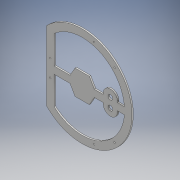
# Autodesk Inventor part: Top Plate1
Saved by Autodesk Inventor 2018 (Build 220112000, 112)
## iProperties
Created: 2017-10-19
Part Number: Top Plate1
Material: Generic
Document SubType Name: Modeling
Designer: BrisbaneMatt
Density: 1 g/cm^3
Appearance: Default
Author: BrisbaneMatt
Autodesk Inventor part; units mm, degrees
ref_plane "YZ Plane" through (0, 0, 0) normal (1, 0, 0) x (0, 1, 0)
ref_plane "XZ Plane" through (0, 0, 0) normal (0, 1, 0) x (-1, 0, 0)
ref_plane "XY Plane" through (0, 0, 0) normal (0, 0, 1) x (1, 0, 0)
sketch "Sketch1" plane through (0, 0, 0) normal (0, 1, 0) x (-1, 0, 0)
  circle A0 centre (0, 0) radius 105
  line L0 (105, 0) -> (75, 0)
  line L1 (75, 0) -> (75, -73.4847)
  line L2 (75, 0) -> (75, 73.4847)
  dimension "d0" = 210
  dimension "d1" = 30
  constraints: 6 end point, 3 point on circle, 1 centre point, 1 coincident, 1 horizontal, 1 perpendicular, 1 point on line
  measures "d0" diameter of A0
  measures "d1" distance of L0.start L0.end
extrude "Extrusion1" add sketch "Sketch1" along normal blind 3 contours L2 L1 A0
sketch "Sketch2" plane through (0, 3, 0) normal (0, 1, 0) x (1, 0, 0)
  line L0 (-75, 73.4847) -> (-75, -73.4847) projected
  line L1 (-75, 0) -> (-67.25, 0)
  line L2 (-67.25, 0) -> (-67.25, -52.6096)
  line L3 (-67.25, -52.6096) -> (-67.25, 59.9001)
  line L4 (0, 0) -> (-67.25, -18.0196)
  line L5 (0, 0) -> (69.6223, 0) construction
  line L6 (0, 0) -> (-67.25, 18.0196)
  line L7 (0, 0) -> (69.6223, 0) construction
  line L8 (0, 0) -> (25.0407, -93.4533)
  line L9 (0, 0) -> (96.75, 0) construction
  line L10 (0, 0) -> (68.4126, -68.4126)
  line L11 (0, 0) -> (96.75, 0) construction
  line L12 (0, 0) -> (25.0407, 93.4533)
  line L13 (0, 0) -> (96.75, 0) construction
  line L14 (0, 0) -> (68.4126, 68.4126)
  line L15 (0, 0) -> (96.75, 0) construction
  circle A0 centre (-67.25, 18.0196) radius 1.5
  circle A1 centre (-67.25, -18.0196) radius 1.5
  circle A2 centre (25.0407, 93.4533) radius 1.5
  circle A3 centre (68.4126, 68.4126) radius 1.5
  circle A4 centre (68.4126, -68.4126) radius 1.5
  circle A5 centre (25.0407, -93.4533) radius 1.5
  dimension "d4" = 7.75
  dimension "d5" = 165
  dimension "d6" = 165
  dimension "d7" = 96.75
  dimension "d8" = 75
  dimension "d9" = 96.75
  dimension "d10" = 45
  dimension "d11" = 96.75
  dimension "d12" = 75
  dimension "d13" = 96.75
  dimension "d14" = 45
  dimension "d15" = 3
  dimension "d16" = 3
  dimension "d17" = 3
  dimension "d18" = 3
  dimension "d19" = 3
  dimension "d20" = 3
  constraints: 30 end point, 7 horizontal, 6 centre point, 6 coincident, 6 equal length, 3 perpendicular, 3 point on line, 1 midpoint
  measures "d4" distance of L1.start L1.end
  measures "d5" angle of L4 L5
  measures "d6" angle of L7 L6
  measures "d7" distance of L4.start L8.end
  measures "d8" angle of L8 L9
  measures "d9" distance of L4.start L10.end
  measures "d10" angle of L10 L11
  measures "d11" distance of L4.start L12.end
  measures "d12" angle of L13 L12
  measures "d13" distance of L4.start L14.end
  measures "d14" angle of L15 L14
  measures "d15" diameter of A0
  measures "d16" diameter of A1
  measures "d17" diameter of A2
  measures "d18" diameter of A3
  measures "d19" diameter of A4
  measures "d20" diameter of A5
extrude "Extrusion2" cut sketch "Sketch2" against normal blind 3 contours A1 L4 L2 | L2 A1 | A0 L3 | L3 L6 A0 | L4 A1 L2 | L3 A0 L6 | A2 | A3 | A4 | A5
sketch "Sketch3" plane through (0, 3, 0) normal (0, 1, 0) x (1, 0, 0)
  circle A0 centre (-67.25, -18.0196) radius 1.5 projected
  line L0 (-67.25, -18.0196) -> (-75, -18.0196)
  line L1 (-75, 73.4847) -> (-75, -73.4847) projected
  line L2 (-75, -18.0196) -> (-59.5, -18.0196)
  line L3 (-59.5, -18.0196) -> (-59.5, -66.8581)
  line L4 (-59.5, -18.0196) -> (-59.5, 66.8581)
  arc A1 (-59.5, -66.8581) -> (-59.5, 66.8581) centre (0, 0) ccw
  point P0 (0, 0)
  dimension "d23" = 15.5
  constraints: 8 end point, 3 point on line, 2 point on circle, 1 centre point, 1 horizontal, 1 vertical
  measures "d23" distance of L0.end L2.end
extrude "Extrusion3" cut sketch "Sketch3" against normal blind 3 contours L4 A1 L3
sketch "Sketch4" plane through (0, 3, 0) normal (0, 1, 0) x (1, 0, 0)
  arc A0 (-59.5, -66.8581) -> (-59.5, 66.8581) centre (0, 0) ccw projected
  line L0 (89.5, 0) -> (59.5, 0)
  line L1 (59.5, 0) -> (59.5, 10)
  line L2 (59.5, 10) -> (59.5, -10)
  circle A1 centre (59.5, -10) radius 5
  circle A2 centre (59.5, 10) radius 5
  circle A3 centre (59.5, 10) radius 15
  circle A4 centre (59.5, -10) radius 15
  line L3 (44.5, -10) -> (44.5, 10)
  line L4 (74.5, 10) -> (74.5, -10)
  point P0 (0, 0)
  dimension "d27" = 30
  dimension "d28" = 10
  dimension "d29" = 20
  dimension "d30" = 10
  dimension "d31" = 10
  constraints: 10 end point, 5 point on circle, 4 centre point, 4 coincident, 2 tangent, 1 horizontal, 1 parallel, 1 perpendicular, 1 point on line, 1 vertical
  measures "d27" distance of L0.start L0.end
  measures "d28" distance of L0.end L1.end
  measures "d29" distance of L1.end L2.end
  measures "d30" diameter of A1
  measures "d31" diameter of A2
extrude "Extrusion4" add sketch "Sketch4" against normal blind 3
sketch "Sketch5" plane through (0, 3, 0) normal (0, 1, 0) x (1, 0, 0)
  line L0 (44.5, -10) -> (44.5, 10) projected
  line L1 (44.5, 0) -> (-59.5, 0)
  line L2 (-59.5, 66.8581) -> (-59.5, -66.8581) projected
  line L3 (-41.4459, 0) -> (-41.4459, 7.5)
  line L4 (-41.4459, 7.5) -> (-41.4459, -7.5)
  line L5 (-41.4459, -7.5) -> (-59.5, -7.5)
  line L6 (-41.4459, -7.5) -> (44.5, -7.5)
  line L7 (-41.4459, 7.5) -> (-59.5, 7.5)
  line L8 (-41.4459, 7.5) -> (44.5, 7.5)
  point P0 (0, 0)
  dimension "d34" = 7.5
  dimension "d35" = 15
  constraints: 14 end point, 7 point on line, 3 perpendicular, 2 midpoint
  measures "d34" distance of L3.start L3.end
  measures "d35" distance of L3.end L4.end
extrude "Extrusion5" add sketch "Sketch5" against normal blind 3 contours L1 L3 L8 L0 | L5 L2 L1 L4 | L1 L2 L7 L3
sketch "Sketch6" plane through (0, 3, 0) normal (0, 1, 0) x (1, 0, 0)
  line L0 (-41.4459, -7.5) -> (-41.4459, 0) projected
  line L1 (-41.4459, 0) -> (44.5, 0) projected
  line L2 (-41.4459, -7.5) -> (44.5, -7.5)
  line L3 (44.5, -7.5) -> (44.5, 0)
  line L4 (44.5, 0) -> (-41.4459, 0)
  line L5 (-41.4459, 0) -> (-41.4459, -7.5)
  point P0 (0, 0)
  constraints: 8 end point, 2 parallel, 1 horizontal, 1 perpendicular
extrude "Extrusion6" add sketch "Sketch6" against normal blind 3
sketch "Sketch7" plane through (0, 3, 0) normal (0, 1, 0) x (1, 0, 0)
  line L0 (44.5, -7.5) -> (-59.5, -7.5) projected
  line L1 (74.5, 10) -> (74.5, -10) projected
  line L2 (44.5, -7.5) -> (74.5, -7.5)
  line L3 (74.5, -7.5) -> (74.5, 7.5)
  line L4 (74.5, 7.5) -> (44.5, 7.5)
  line L5 (44.5, 7.5) -> (44.5, -7.5)
  line L6 (74.5, 7.5) -> (92.1337, 7.5)
  line L7 (92.1337, 7.5) -> (92.1337, -7.5)
  line L8 (92.1337, -7.5) -> (74.5, -7.5)
  line L9 (74.5, -7.5) -> (74.5, 7.5)
  point P0 (0, 0)
  dimension "d40" = 15
  constraints: 16 end point, 4 parallel, 2 horizontal, 2 perpendicular, 2 point on line
  measures "d40" distance of L3.end L2.end
extrude "Extrusion7" add sketch "Sketch7" against normal blind 3 contours L6 L7 L8 L1
sketch "Sketch8" plane through (0, 3, 0) normal (0, 1, 0) x (1, 0, 0)
  line L0 (0, 0) -> (-30, 0)
  line L1 (0, 0) -> (-15, 25.9808)
  line L2 (0, 0) -> (30, 0) construction
  line L3 (-15, 25.9808) -> (-30, 0)
  line L4 (0, 0) -> (15, 25.9808)
  line L5 (15, 25.9808) -> (-15, 25.9808)
  line L6 (0, 0) -> (30, 0)
  line L7 (30, 0) -> (15, 25.9808)
  line L8 (0, 0) -> (15, -25.9808)
  line L9 (15, -25.9808) -> (30, 0)
  line L10 (0, 0) -> (-15, -25.9808)
  line L11 (-15, -25.9808) -> (15, -25.9808)
  line L12 (-15, -25.9808) -> (-30, 0)
  dimension "d43" = 30
  dimension "d44" = 30
  dimension "d45" = 120
  constraints: 26 end point, 5 horizontal, 5 parallel, 1 equal length, 1 point on line
  measures "d43" distance of L0.start L0.end
  measures "d44" distance of L0.start L1.end
  measures "d45" angle of L2 L1
extrude "Extrusion8" add sketch "Sketch8" against normal blind 3 contours L10 L12 L0 | L0 L3 L1 | L4 L7 L6 | L6 L9 L8 | L8 L11 L10
sketch "Sketch9" plane through (0, 3, 0) normal (0, 1, 0) x (1, 0, 0)
  line L0 (4.3301, 7.5) -> (15, 25.9808) projected
  line L1 (-25.6699, 7.5) -> (-15, 25.9808) projected
  line L2 (15, 25.9808) -> (-15, 25.9808)
  line L3 (-15, 25.9808) -> (-4.3301, 7.5) projected
  line L4 (-15, 25.9808) -> (-4.3301, 7.5)
  line L5 (-4.3301, 7.5) -> (4.3988, 7.5)
  line L6 (-4.3301, 7.5) -> (4.3301, 7.5) projected
  line L7 (25.6699, 7.5) -> (15, 25.9808) projected
  line L8 (4.3301, 7.5) -> (15, 25.9808)
  point P0 (0, 0)
  constraints: 8 end point, 1 collinear, 1 horizontal, 1 parallel
extrude "Extrusion9" add sketch "Sketch9" against normal blind 3
body "Solid1"
